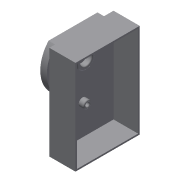
# Autodesk Inventor part: GearHolder
Saved by Autodesk Inventor 2018 (Build 220112000, 112)
## iProperties
Created: 2018-10-25
Part Number: GearHolder
Material: Generic
Document SubType Name: Modeling
Designer: Vulnic
Density: 1 g/cm^3
Appearance: Default
Author: Vulnic
Autodesk Inventor part; units mm, degrees
ref_plane "YZ Plane" through (0, 0, 0) normal (1, 0, 0) x (0, 1, 0)
ref_plane "XZ Plane" through (0, 0, 0) normal (0, 1, 0) x (-1, 0, 0)
ref_plane "XY Plane" through (0, 0, 0) normal (0, 0, 1) x (1, 0, 0)
sketch "Sketch1" plane through (0, 0, 0) normal (1, 0, 0) x (0, 1, 0)
  circle A0 centre (3.7472, 31.8344) radius 0.7 projected
  arc A1 (6.295, 21.1336) -> (6.4355, 23.5076) centre (-1.824, 22.8051) ccw projected
  arc A2 (5.4476, 20.9667) -> (6.295, 21.1336) centre (3.7472, 31.8344) ccw projected
  arc A3 (4.4173, 23.1101) -> (5.4476, 20.9667) centre (12.3263, 25.5922) ccw projected
  arc A4 (3.7308, 23.0845) -> (4.4173, 23.1101) centre (3.7472, 31.8344) ccw projected
  arc A5 (2.8636, 20.87) -> (3.7308, 23.0845) centre (-4.3415, 24.9686) ccw projected
  arc A6 (2.006, 20.9731) -> (2.8636, 20.87) centre (3.7472, 31.8344) ccw projected
  arc A7 (1.6886, 23.33) -> (2.006, 20.9731) centre (9.9774, 23.2466) ccw projected
  arc A8 (1.0277, 23.5178) -> (1.6886, 23.33) centre (3.7472, 31.8344) ccw projected
  arc A9 (-0.4814, 21.6797) -> (1.0277, 23.5178) centre (-6.0673, 27.8042) ccw projected
  arc A10 (-1.2651, 22.0427) -> (-0.4814, 21.6797) centre (3.7472, 31.8344) ccw projected
  arc A11 (-0.8387, 24.3824) -> (-1.2651, 22.0427) centre (7.0187, 21.7417) ccw projected
  arc A12 (-1.4092, 24.7652) -> (-0.8387, 24.3824) centre (3.7472, 31.8344) ccw projected
  arc A13 (-3.4124, 23.4834) -> (-1.4092, 24.7652) centre (-6.8324, 31.0342) ccw projected
  arc A14 (-4.0456, 24.0709) -> (-3.4124, 23.4834) centre (3.7472, 31.8344) ccw projected
  arc A15 (-2.917, 26.1642) -> (-4.0456, 24.0709) centre (3.7397, 21.2247) ccw projected
  arc A16 (-3.3414, 26.7046) -> (-2.917, 26.1642) centre (3.7472, 31.8344) ccw projected
  arc A17 (-5.6426, 26.1045) -> (-3.3414, 26.7046) centre (-6.5618, 34.3427) ccw projected
  arc A18 (-6.0632, 26.8589) -> (-5.6426, 26.1045) centre (3.7472, 31.8344) ccw projected
  arc A19 (-4.343, 28.5011) -> (-6.0632, 26.8589) centre (0.4615, 21.7463) ccw projected
  arc A20 (-4.5796, 29.1461) -> (-4.343, 28.5011) centre (3.7472, 31.8344) ccw projected
  arc A21 (-6.9537, 29.2866) -> (-4.5796, 29.1461) centre (-5.2822, 37.4056) ccw projected
  arc A22 (-7.1206, 30.134) -> (-6.9537, 29.2866) centre (3.7472, 31.8344) ccw projected
  arc A23 (-4.9771, 31.1643) -> (-7.1206, 30.134) centre (-2.4951, 23.2553) ccw projected
  arc A24 (-5.0028, 31.8508) -> (-4.9771, 31.1643) centre (3.7472, 31.8344) ccw projected
  arc A25 (-7.2173, 32.718) -> (-5.0028, 31.8508) centre (-3.1187, 39.9231) ccw projected
  arc A26 (-7.1142, 33.5756) -> (-7.2173, 32.718) centre (3.7472, 31.8344) ccw projected
  arc A27 (-4.7572, 33.893) -> (-7.1142, 33.5756) centre (-4.8407, 25.6042) ccw projected
  arc A28 (-4.5695, 34.5539) -> (-4.7572, 33.893) centre (3.7472, 31.8344) ccw projected
  arc A29 (-6.4076, 36.063) -> (-4.5695, 34.5539) centre (-0.2831, 41.6489) ccw projected
  arc A30 (-6.0445, 36.8467) -> (-6.4076, 36.063) centre (3.7472, 31.8344) ccw projected
  arc A31 (-3.7048, 36.4203) -> (-6.0445, 36.8467) centre (-6.3456, 28.5629) ccw projected
  arc A32 (-3.3221, 36.9908) -> (-3.7048, 36.4203) centre (3.7472, 31.8344) ccw projected
  arc A33 (-4.6039, 38.994) -> (-3.3221, 36.9908) centre (2.947, 42.414) ccw projected
  arc A34 (-4.0164, 39.6272) -> (-4.6039, 38.994) centre (3.7472, 31.8344) ccw projected
  arc A35 (-1.923, 38.4986) -> (-4.0164, 39.6272) centre (-6.8626, 31.8419) ccw projected
  arc A36 (-1.3827, 38.923) -> (-1.923, 38.4986) centre (3.7472, 31.8344) ccw projected
  arc A37 (-1.9827, 41.2242) -> (-1.3827, 38.923) centre (6.2554, 42.1434) ccw projected
  arc A38 (-1.2283, 41.6448) -> (-1.9827, 41.2242) centre (3.7472, 31.8344) ccw projected
  arc A39 (0.4139, 39.9246) -> (-1.2283, 41.6448) centre (-6.341, 35.1201) ccw projected
  arc A40 (1.0589, 40.1612) -> (0.4139, 39.9246) centre (3.7472, 31.8344) ccw projected
  arc A41 (1.1993, 42.5353) -> (1.0589, 40.1612) centre (9.3183, 40.8638) ccw projected
  arc A42 (2.0468, 42.7022) -> (1.1993, 42.5353) centre (3.7472, 31.8344) ccw projected
  arc A43 (3.077, 40.5587) -> (2.0468, 42.7022) centre (-4.8319, 38.0767) ccw projected
  arc A44 (3.7636, 40.5844) -> (3.077, 40.5587) centre (3.7472, 31.8344) ccw projected
  arc A45 (4.6308, 42.7989) -> (3.7636, 40.5844) centre (11.8359, 38.7003) ccw projected
  arc A46 (5.4883, 42.6958) -> (4.6308, 42.7989) centre (3.7472, 31.8344) ccw projected
  arc A47 (5.8058, 40.3388) -> (5.4883, 42.6958) centre (-2.4831, 40.4223) ccw projected
  arc A48 (6.4667, 40.1511) -> (5.8058, 40.3388) centre (3.7472, 31.8344) ccw projected
  arc A49 (7.9757, 41.9892) -> (6.4667, 40.1511) centre (13.5616, 35.8647) ccw projected
  arc A50 (8.7594, 41.6261) -> (7.9757, 41.9892) centre (3.7472, 31.8344) ccw projected
  arc A51 (8.333, 39.2865) -> (8.7594, 41.6261) centre (0.4756, 41.9272) ccw projected
  arc A52 (8.9036, 38.9037) -> (8.333, 39.2865) centre (3.7472, 31.8344) ccw projected
  arc A53 (10.9068, 40.1855) -> (8.9036, 38.9037) centre (14.3267, 32.6346) ccw projected
  arc A54 (11.5399, 39.598) -> (10.9068, 40.1855) centre (3.7472, 31.8344) ccw projected
  arc A55 (10.4114, 37.5046) -> (11.5399, 39.598) centre (3.7546, 42.4442) ccw projected
  arc A56 (10.8357, 36.9643) -> (10.4114, 37.5046) centre (3.7472, 31.8344) ccw projected
  arc A57 (13.137, 37.5643) -> (10.8357, 36.9643) centre (14.0562, 29.3262) ccw projected
  arc A58 (13.5576, 36.81) -> (13.137, 37.5643) centre (3.7472, 31.8344) ccw projected
  arc A59 (11.8374, 35.1678) -> (13.5576, 36.81) centre (7.0328, 41.9226) ccw projected
  arc A60 (12.074, 34.5227) -> (11.8374, 35.1678) centre (3.7472, 31.8344) ccw projected
  arc A61 (14.448, 34.3823) -> (12.074, 34.5227) centre (12.7765, 26.2633) ccw projected
  arc A62 (14.615, 33.5348) -> (14.448, 34.3823) centre (3.7472, 31.8344) ccw projected
  arc A63 (12.4715, 32.5046) -> (14.615, 33.5348) centre (9.9894, 40.4135) ccw projected
  arc A64 (12.4972, 31.818) -> (12.4715, 32.5046) centre (3.7472, 31.8344) ccw projected
  arc A65 (14.7116, 30.9508) -> (12.4972, 31.818) centre (10.613, 23.7458) ccw projected
  arc A66 (14.6085, 30.0933) -> (14.7116, 30.9508) centre (3.7472, 31.8344) ccw projected
  arc A67 (12.2516, 29.7758) -> (14.6085, 30.0933) centre (12.335, 38.0647) ccw projected
  arc A68 (12.0638, 29.1149) -> (12.2516, 29.7758) centre (3.7472, 31.8344) ccw projected
  arc A69 (13.9019, 27.6059) -> (12.0638, 29.1149) centre (7.7775, 22.02) ccw projected
  arc A70 (13.5389, 26.8222) -> (13.9019, 27.6059) centre (3.7472, 31.8344) ccw projected
  arc A71 (11.1992, 27.2486) -> (13.5389, 26.8222) centre (13.8399, 35.106) ccw projected
  arc A72 (10.8164, 26.6781) -> (11.1992, 27.2486) centre (3.7472, 31.8344) ccw projected
  arc A73 (12.0982, 24.6748) -> (10.8164, 26.6781) centre (4.5474, 21.2549) ccw projected
  arc A74 (11.5108, 24.0417) -> (12.0982, 24.6748) centre (3.7472, 31.8344) ccw projected
  arc A75 (9.4174, 25.1702) -> (11.5108, 24.0417) centre (14.3569, 31.827) ccw projected
  arc A76 (8.877, 24.7459) -> (9.4174, 25.1702) centre (3.7472, 31.8344) ccw projected
  arc A77 (9.4771, 22.4446) -> (8.877, 24.7459) centre (1.2389, 21.5254) ccw projected
  arc A78 (8.7227, 22.024) -> (9.4771, 22.4446) centre (3.7472, 31.8344) ccw projected
  arc A79 (7.0805, 23.7442) -> (8.7227, 22.024) centre (13.8353, 28.5488) ccw projected
  arc A80 (6.4355, 23.5076) -> (7.0805, 23.7442) centre (3.7472, 31.8344) ccw projected
  line L0 (4.9954, 45.8746) -> (4.8965, 48.5188) projected
  arc A81 (4.8965, 48.5188) -> (4.9954, 45.8746) centre (3.1894, 47.131) ccw projected
  arc A82 (-0.8751, 51.5446) -> (0.2488, 49.4581) centre (4.3942, 53.0372) ccw projected
  arc A83 (-0.1346, 52.1261) -> (-0.8751, 51.5446) centre (3.1894, 47.131) ccw projected
  arc A84 (1.6258, 50.5395) -> (-0.1346, 52.1261) centre (-2.834, 47.3609) ccw projected
  arc A85 (2.1783, 50.7421) -> (1.6258, 50.5395) centre (3.1894, 47.131) ccw projected
  arc A86 (2.4954, 53.0907) -> (2.1783, 50.7421) centre (7.6357, 51.201) ccw projected
  arc A87 (3.4362, 53.1259) -> (2.4954, 53.0907) centre (3.1894, 47.131) ccw projected
  arc A88 (3.9279, 50.8076) -> (3.4362, 53.1259) centre (-1.5485, 50.8574) ccw projected
  arc A89 (4.4939, 50.6468) -> (3.9279, 50.8076) centre (3.1894, 47.131) ccw projected
  arc A90 (6.131, 52.3605) -> (4.4939, 50.6468) centre (9.1788, 47.8103) ccw projected
  arc A91 (6.9128, 51.8359) -> (6.131, 52.3605) centre (3.1894, 47.131) ccw projected
  arc A92 (5.9479, 49.6713) -> (6.9128, 51.8359) centre (1.5467, 52.9306) ccw projected
  arc A93 (6.3113, 49.2085) -> (5.9479, 49.6713) centre (3.1894, 47.131) ccw projected
  arc A94 (8.643, 49.6327) -> (6.3113, 49.2085) centre (8.4342, 44.1601) ccw projected
  arc A95 (8.9672, 48.7488) -> (8.643, 49.6327) centre (3.1894, 47.131) ccw projected
  arc A96 (6.9142, 47.5648) -> (8.9672, 48.7488) centre (5.2694, 52.7886) ccw projected
  arc A97 (6.9362, 46.9768) -> (6.9142, 47.5648) centre (3.1894, 47.131) ccw projected
  arc A98 (9.0719, 45.9494) -> (6.9362, 46.9768) centre (5.6863, 41.6447) ccw projected
  arc A99 (8.8147, 45.0438) -> (9.0719, 45.9494) centre (3.1894, 47.131) ccw projected
  arc A100 (6.4578, 45.2925) -> (8.8147, 45.0438) centre (8.1976, 50.4855) ccw projected
  arc A101 (6.13, 44.8039) -> (6.4578, 45.2925) centre (3.1894, 47.131) ccw projected
  arc A102 (7.254, 42.7174) -> (6.13, 44.8039) centre (1.9846, 41.2248) ccw projected
  arc A103 (6.5135, 42.1359) -> (7.254, 42.7174) centre (3.1894, 47.131) ccw projected
  arc A104 (4.753, 43.7225) -> (6.5135, 42.1359) centre (9.2128, 46.9012) ccw projected
  arc A105 (4.2006, 43.5199) -> (4.753, 43.7225) centre (3.1894, 47.131) ccw projected
  arc A106 (3.8835, 41.1713) -> (4.2006, 43.5199) centre (-1.2568, 43.061) ccw projected
  arc A107 (2.9426, 41.1361) -> (3.8835, 41.1713) centre (3.1894, 47.131) ccw projected
  arc A108 (2.4509, 43.4544) -> (2.9426, 41.1361) centre (7.9274, 43.4046) ccw projected
  arc A109 (1.8849, 43.6152) -> (2.4509, 43.4544) centre (3.1894, 47.131) ccw projected
  arc A110 (0.2479, 41.9015) -> (1.8849, 43.6152) centre (-2.8, 46.4517) ccw projected
  arc A111 (-0.534, 42.4261) -> (0.2479, 41.9015) centre (3.1894, 47.131) ccw projected
  arc A112 (0.4309, 44.5907) -> (-0.534, 42.4261) centre (4.8322, 41.3314) ccw projected
  arc A113 (0.0675, 45.0535) -> (0.4309, 44.5907) centre (3.1894, 47.131) ccw projected
  arc A114 (-2.2641, 44.6293) -> (0.0675, 45.0535) centre (-2.0554, 50.1019) ccw projected
  arc A115 (-2.5884, 45.5132) -> (-2.2641, 44.6293) centre (3.1894, 47.131) ccw projected
  arc A116 (-0.5354, 46.6972) -> (-2.5884, 45.5132) centre (1.1095, 41.4734) ccw projected
  arc A117 (-0.5574, 47.2852) -> (-0.5354, 46.6972) centre (3.1894, 47.131) ccw projected
  arc A118 (-2.6931, 48.3126) -> (-0.5574, 47.2852) centre (0.6926, 52.6173) ccw projected
  arc A119 (-2.4358, 49.2183) -> (-2.6931, 48.3126) centre (3.1894, 47.131) ccw projected
  arc A120 (-0.079, 48.9695) -> (-2.4358, 49.2183) centre (-1.8187, 43.7765) ccw projected
  arc A121 (0.2488, 49.4581) -> (-0.079, 48.9695) centre (3.1894, 47.131) ccw projected
  line L1 (16.152, 19.5075) -> (-8.3796, 19.5075)
  line L2 (-8.3796, 19.5075) -> (-8.3796, 55.4678)
  line L3 (-8.3796, 55.4678) -> (16.152, 55.4678)
  line L4 (16.152, 55.4678) -> (16.152, 19.5075)
  point P0 (0, 0)
  constraints: 8 end point, 2 parallel, 1 horizontal, 1 perpendicular
extrude "Extrusion1" add sketch "Sketch1" along normal blind 10 contours A0 | A2 A3 A4 A5 A6 A7 A8 A9 A10 A11 A12 A13 A14 A15 A16 A17 A18 A19 A20 A21 A22 A23 A24 A25 A26 A27 A28 A29 A30 A31 A32 A33 A34 A35 A36 A37 A38 A39 A40 A41 A42 A43 A44 A45 A46 A47 A48 A49 A50 A51 A52 A53 A54 A55 A56 A57 A58 A59 A60 A61 A62 A63 A64 A65 A66 A67 A68 A69 A70 A71 A72 A73 A74 A75 A76 A77 A78 A79 A80 A1 | A81 L0 | A83 A84 A85 A86 A87 A88 A89 A90 A91 A92 A93 A94 A95 A96 A97 A98 A99 A100 A101 A102 A103 A104 A105 A106 A107 A108 A109 A110 A111 A112 A113 A114 A115 A116 A117 A118 A119 A120 A121 A82 | L1 L2 L3 L4
shell "Shell1" thickness 0.6 removed faces 1 at (10, -0.2024, 43.481)
sketch "Sketch3" plane through (0.6, -7.7796, 20.1075) normal (1, 0, 0) x (0, 0, -1)
  circle A0 centre (-11.7269, 11.5268) radius 0.8
  circle A1 centre (-27.0563, 10.9578) radius 3.5 projected
  circle A2 centre (-11.7269, 11.5268) radius 1.5
  circle A3 centre (-27.0235, 10.969) radius 2.4
  point P0 (20.1075, 7.7796)
  dimension "d3" = 3
  dimension "d19" = 4.8
  dimension "d20" = 1.6
  constraints: 3 centre point, 1 coincident
  measures "d3" diameter of A2
  measures "d19" diameter of A3
  measures "d20" diameter of A0
extrude "Extrusion3" add sketch "Sketch3" along normal blind 2
fillet "Fillet1" radius 0.2 4 edges at (2.6, 3.1894, 49.531) (2.6, 3.1782, 50.6638) (2.6, 3.7472, 32.6344) (2.6, 3.7472, 33.3344)
sketch "Sketch4" plane through (0, 0, 0) normal (-1, 0, 0) x (0, 0, 1)
  circle A0 centre (47.1638, -5.3218) radius 1.45
  circle A1 centre (47.1638, 11.6782) radius 1.45
  point P0 (0, 0)
  dimension "d13" = 2.9
  dimension "d14" = 2.9
  constraints: 2 centre point, 2 other
  measures "d13" diameter of A1
  measures "d14" diameter of A0
extrude "Extrusion4" cut sketch "Sketch4" against normal through all
sketch "Sketch5" plane through (0, 0, 0) normal (-1, 0, 0) x (0, 0, 1)
  circle A0 centre (47.1638, 3.1782) radius 3.5
  circle A1 centre (47.1638, 3.1782) radius 12.5
  circle A2 centre (47.1638, 11.6782) radius 1.45 projected
  circle A3 centre (47.1638, -5.3218) radius 1.25
  line L0 (55.4678, -8.3796) -> (55.4678, 16.152) projected
  line L1 (55.4678, -6.1649) -> (55.4678, 12.5213)
  point P0 (0, 0)
  constraints: 3 centre point, 2 end point, 2 point on circle, 2 point on line, 6 other
extrude "Extrusion5" add sketch "Sketch5" along normal blind 2.5 contours L0 A1 picked at (53.8665, 3.1782)
sketch "Sketch7" plane through (-2.5, 0, 0) normal (-1, 0, 0) x (0, 0, 1)
  circle A0 centre (47.1638, 3.1782) radius 3.5 projected
  circle A1 centre (47.131, 3.1894) radius 2.4 projected
  point P0 (0, 0)
extrude "Extrusion7" cut sketch "Sketch7" against normal through all contours A1
sketch "Sketch8" plane through (-2.5, 0, 0) normal (-1, 0, 0) x (0, 0, 1)
  circle A0 centre (47.1638, -5.3218) radius 1.45 projected
  point P0 (0, 0)
extrude "Extrusion8" cut sketch "Sketch8" against normal through all
body "Solid1"
